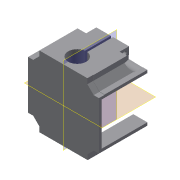
# Autodesk Inventor part: 20_Cube_insert_AlliedVision_Alvium_v3
Saved by Autodesk Inventor 2022 (Build 260153000, 153)
## iProperties
Created: 2019-08-07
Part Number: 20_Cube_insert_AlliedVision_Alvium_v3
Material: Generic
Document SubType Name: Modeling
Designer: marsikovabarbora
Density: 1 g/cm^3
Appearance: Default
Sheet Metal Rule: Standard
Author: marsikovabarbora
Autodesk Inventor part; units mm, degrees
ref_plane "Work Plane1" through (-29.1, -14.5, 2.4) normal (0, 0, -1) x (0, 1, 0)
ref_plane "Work Plane2" through (-13.8999, -10.5497, 2.25) normal (0, 0, -1) x (0, 1, 0)
ref_plane "Work Plane4" through (-17.3325, -17.0101, 2.3331) normal (0.0023441, 0.0023441, -0.9999945) x (-0.0000027, 0.9999973, 0.0023441)
sketch "Sketch1" plane through (0, 0, 0) normal (0, 0, 1) x (1, 0, 0)
  line L0 (-34.86, 0) -> (34.86, 0) construction
  line L1 (0, -34.86) -> (0, 34.86) construction
  line L2 (0, 0) -> (11.1575, 11.1575) construction
  line L3 (0, 0) -> (15.7791, 0) construction
  line L4 (0, 24.9) -> (16.8009, 24.9)
  line L5 (16.8009, 24.9) -> (16.8009, 21.2415)
  line L6 (16.8009, 21.2415) -> (19.0212, 19.0212)
  line L7 (24.9, 0) -> (24.9, 16.8009)
  line L8 (24.9, 16.8009) -> (21.2415, 16.8009)
  line L9 (21.2415, 16.8009) -> (19.0212, 19.0212)
  line L10 (0, -24.9) -> (16.8009, -24.9)
  line L11 (16.8009, -24.9) -> (16.8009, -21.2415)
  line L12 (16.8009, -21.2415) -> (19.0212, -19.0212)
  line L13 (24.9, 0) -> (24.9, -16.8009)
  line L14 (24.9, -16.8009) -> (21.2415, -16.8009)
  line L15 (21.2415, -16.8009) -> (19.0212, -19.0212)
  line L16 (0, 24.9) -> (-16.8009, 24.9)
  line L17 (-16.8009, 24.9) -> (-16.8009, 21.2415)
  line L18 (-16.8009, 21.2415) -> (-19.0212, 19.0212)
  line L19 (-24.9, 16.8009) -> (-21.2415, 16.8009)
  line L20 (-21.2415, 16.8009) -> (-19.0212, 19.0212)
  line L21 (0, -24.9) -> (-16.8009, -24.9)
  line L22 (-16.8009, -24.9) -> (-16.8009, -21.2415)
  line L23 (-16.8009, -21.2415) -> (-19.0212, -19.0212)
  line L24 (-21.2415, -16.8009) -> (-19.0212, -19.0212)
  line L25 (-24.9, -16.8009) -> (-21.2415, -16.8009)
  line L26 (-24.9, 0) -> (-24.9, -16.8009)
  line L27 (-24.9, 0) -> (-24.9, 16.8009)
  circle A0 centre (0, 0) radius 10
  dimension "d0" = 45
  dimension "d2" = 24.9
  dimension "d3" = 3.14
  dimension "d4" = 26.9
  dimension "d5" = 20
  constraints: 52 end point, 20 symmetric about line, 2 horizontal, 2 perpendicular, 2 point on line, 1 centre point, 1 coincident, 1 equal length
  measures "d0" angle of L3 L2
  measures "d2" distance between parallel lines of L0 L4
  measures "d3" distance of L5.end L6.end
  measures "d4" distance from line of L2.start L6
  measures "d5" diameter of A0
extrude "Extrusion1" add sketch "Sketch1" along normal blind 4 contours L4 L5 L6 L9 L8 L7 L13 L14 L15 L12 L11 L10 L21 L22 L23 L24 L25 L26 L27 L19 L20 L18 L17 L16 | A0
sketch "Skizze6" plane through (-16.8009, 24.9, 4) normal (0, 0, 1) x (1, 0, 0)
  circle A0 centre (6.8009, -18) radius 1.65 construction
  circle A1 centre (3.0009, -24.9) radius 1.65 construction
  circle A2 centre (26.5009, -34.9) radius 1.65 construction
  circle A3 centre (26.5009, -14.9) radius 1.65 construction
  line L0 (33.6017, -3.6585) -> (33.6017, 0) projected
  line L1 (33.6017, 0) -> (0, 0) construction
  line L2 (0, 0) -> (0, -3.6585) projected
  line L3 (0, -3.6585) -> (-4.4406, -8.0991) projected
  line L4 (-4.4406, -8.0991) -> (-8.0991, -8.0991) projected
  line L5 (-8.0991, -8.0991) -> (-8.0991, -41.7009) construction
  line L6 (-8.0991, -41.7009) -> (-4.4406, -41.7009) projected
  line L7 (-4.4406, -41.7009) -> (0, -46.1415) projected
  line L8 (0, -46.1415) -> (0, -49.8) projected
  line L9 (0, -49.8) -> (33.6017, -49.8) construction
  line L10 (33.6017, -49.8) -> (33.6017, -46.1415) projected
  line L11 (33.6017, -46.1415) -> (38.0423, -41.7009) projected
  line L12 (38.0423, -41.7009) -> (41.7009, -41.7009) projected
  line L13 (41.7009, -41.7009) -> (41.7009, -8.0991) construction
  line L14 (41.7009, -8.0991) -> (38.0423, -8.0991) projected
  line L15 (38.0423, -8.0991) -> (33.6017, -3.6585) projected
  line L16 (-0.2, 0.2) -> (33.8017, 0.2) construction
  line L17 (33.8017, 0.2) -> (33.8017, -3.5757)
  line L18 (33.8017, -3.5757) -> (38.1252, -7.8991)
  line L19 (38.1252, -7.8991) -> (41.9009, -7.8991)
  line L20 (41.9009, -7.8991) -> (41.9009, -41.9009) construction
  line L21 (41.9009, -41.9009) -> (38.1252, -41.9009)
  line L22 (38.1252, -41.9009) -> (33.8017, -46.2243)
  line L23 (33.8017, -46.2243) -> (33.8017, -50)
  line L24 (33.8017, -50) -> (-0.2, -50) construction
  line L25 (-0.2, -50) -> (-0.2, -46.2243)
  line L26 (-0.2, -46.2243) -> (-4.5235, -41.9009)
  line L27 (-4.5235, -41.9009) -> (-8.2991, -41.9009)
  line L28 (-8.2991, -41.9009) -> (-8.2991, -7.8991) construction
  line L29 (-8.2991, -7.8991) -> (-4.5235, -7.8991)
  line L30 (-4.5235, -7.8991) -> (-0.2, -3.5757)
  line L31 (-0.2, -3.5757) -> (-0.2, 0.2)
  line L32 (-8.0991, -8.0991) -> (-8.0991, -7.8991)
  line L33 (0, 0) -> (-0.2, 0)
  line L34 (33.6017, 0) -> (33.8017, 0)
  line L35 (41.7009, -8.0991) -> (38.0423, -8.0991) projected
  line L36 (41.7009, -8.0991) -> (41.7009, -7.8991)
  line L37 (41.7009, -41.7009) -> (41.7009, -41.9009)
  line L38 (33.6017, -49.8) -> (33.8017, -49.8)
  line L39 (-8.0991, -41.7009) -> (-8.0991, -41.9009)
  line L40 (0, -49.8) -> (-0.2, -49.8)
  point P0 (16.8009, -24.9)
  dimension "d25" = 0.2
  constraints: 48 end point, 12 point on line, 4 perpendicular, 15 other
  measures "d25" distance between parallel lines of L1 L16
extrude "IM_offset" add sketch "Skizze6" against normal up to surface (4 mm away) contours L2 L3 L4 L32 L29 L30 L31 L33 | L6 L7 L8 L40 L25 L26 L27 L39 | L10 L11 L12 L37 L21 L22 L23 L38
ref_plane "Work Plane3" through (-24.85, -16.97, -31.85) normal (0, 0, 1) x (1, 0, 0)
sketch "Sketch9" plane through (0, 0, 0) normal (0, 0, -1) x (-1, 0, 0)
  line L0 (21.2829, 16.9009) -> (17.0009, 21.2829)
  line L1 (17.0009, 21.2829) -> (17.0009, 24.9)
  line L2 (24.9, 17.0009) -> (21.2829, 16.9009)
  line L3 (24.9, -17.0009) -> (24.9, 17.0009) projected
  line L4 (17.0009, 24.9) -> (-16.8009, 24.9) projected
  line L5 (24.9, 14.96) -> (15.0009, 14.96)
  line L6 (15.0009, 14.96) -> (15.0009, 24.9)
  line L7 (15.0009, 24.9) -> (17.0009, 24.9)
  line L8 (24.9, 17.0009) -> (24.9, 14.96)
  line L9 (-16.9009, 21.2829) -> (-21.2829, 17.0009)
  line L10 (-21.2829, 17.0009) -> (-24.9, 17.0009)
  line L11 (-17.0009, 24.9) -> (-16.9009, 21.2829)
  line L12 (-14.96, 24.9) -> (-14.96, 15.0009)
  line L13 (-14.96, 15.0009) -> (-24.9, 15.0009)
  line L14 (-24.9, 15.0009) -> (-24.9, 17.0009)
  line L15 (-17.0009, 24.9) -> (-14.96, 24.9)
  line L16 (-21.2829, -16.9009) -> (-17.0009, -21.2829)
  line L17 (-17.0009, -21.2829) -> (-17.0009, -24.9)
  line L18 (-24.9, -17.0009) -> (-21.2829, -16.9009)
  line L19 (-24.9, -14.96) -> (-15.0009, -14.96)
  line L20 (-15.0009, -14.96) -> (-15.0009, -24.9)
  line L21 (-15.0009, -24.9) -> (-17.0009, -24.9)
  line L22 (-24.9, -17.0009) -> (-24.9, -14.96)
  line L23 (16.9009, -21.2829) -> (21.2829, -17.0009)
  line L24 (21.2829, -17.0009) -> (24.9, -17.0009)
  line L25 (17.0009, -24.9) -> (16.9009, -21.2829)
  line L26 (14.96, -24.9) -> (14.96, -15.0009)
  line L27 (14.96, -15.0009) -> (24.9, -15.0009)
  line L28 (24.9, -15.0009) -> (24.9, -17.0009)
  line L29 (17.0009, -24.9) -> (14.96, -24.9)
  point P0 (0, 0)
  dimension "d44" = 2
  dimension "d47" = 360
  constraints: 56 end point, 10 point on line, 2 parallel, 1 horizontal, 1 perpendicular, 65 other
  measures "d44" distance of L6.end L7.end
ref_plane "Work Plane5" through (-25.1325, -16.9302, -31.7852) normal (-0.0023441, -0.0023441, 0.9999945) x (0.9999973, -0.0000027, 0.0023441)
ref_plane "Work Plane10" through (-16.97, -16.97, -30.1) normal (0, 0, 1) x (1, 0, 0)
extrude "Extrusion9" add sketch "Sketch9" along normal up to surface (30.1 mm away)
ref_plane "Work Plane6" through (-16.5464, -17.0101, 2.3349) normal (0.0023441, 0.0023441, -0.9999945) x (-0.0000027, 0.9999973, 0.0023441)
sketch "Sketch11" plane through (0, 0, 4) normal (0, 0, 1) x (1, 0, 0)
  circle A0 centre (-10, 6.9) radius 1.65 projected
  circle A1 centre (9.7, 10) radius 1.65 projected
  circle A2 centre (9.7, -10) radius 1.65 projected
  arc A3 (-13.0126, 1.45) -> (-13.0126, -1.45) centre (-13.8, 0) ccw projected
  line L0 (-13.0126, 1.45) -> (15.2888, 1.45) projected
  line L1 (15.2888, -1.45) -> (-13.0126, -1.45) projected
  arc A4 (15.2888, -1.45) -> (15.2888, 1.45) centre (16.0762, 0) ccw projected
  line L2 (16.8009, 24.9) -> (-17.0009, 24.9) projected
  line L3 (-17.0009, 24.9) -> (-17.0009, 21.3243) projected
  line L4 (-17.0009, 21.3243) -> (-21.3243, 17.0009) projected
  line L5 (-21.3243, 17.0009) -> (-24.9, 17.0009) projected
  line L6 (-24.9, 17.0009) -> (-24.9, -17.0009) projected
  line L7 (-24.9, -17.0009) -> (-21.3243, -17.0009) projected
  line L8 (-21.3243, -17.0009) -> (-17.0009, -21.3243) projected
  line L9 (-17.0009, -21.3243) -> (-17.0009, -24.9) projected
  line L10 (-17.0009, -24.9) -> (17.0009, -24.9) projected
  line L11 (17.0009, -24.9) -> (17.0009, -21.3243) projected
  line L12 (17.0009, -21.3243) -> (21.3243, -17.0009) projected
  line L13 (21.3243, -17.0009) -> (24.9, -17.0009) projected
  line L14 (24.9, -17.0009) -> (24.9, 16.8009) projected
  line L15 (24.9, 16.8009) -> (21.2415, 16.8009) projected
  line L16 (21.2415, 16.8009) -> (16.8009, 21.2415) projected
  line L17 (16.8009, 21.2415) -> (16.8009, 24.9) projected
  point P0 (0, 0)
ref_plane "Work Plane7" through (-24.4263, -24.8901, 2.298) normal (0.0023441, 0.0023441, -0.9999945) x (-0.0000027, 0.9999973, 0.0023441)
extrude "Extrusion11" add sketch "Sketch11" against normal up to surface surface through (-24.4263, -24.8901, 2.298) normal (0.0023441, 0.0023441, -0.9999945)
ref_plane "Work Plane8" through (-15.0009, 0, 0) normal (0, 1, 0) x (1, 0, 0)
ref_plane "Work Plane9" through (0, -15.0009, 0) normal (-1, 0, 0) x (0, 0, 1)
sketch "Sketch12" plane through (-24.9, -17.0009, 4) normal (-1, 0, 0) x (0, 0, 1)
  line L0 (0, 34.0017) -> (-4, 34.0017) projected
  line L1 (-4, 34.0017) -> (-34.1, 34.0017) projected
  line L2 (-34.1, 31.9609) -> (-34.1, 34.0017) projected
  line L3 (-4, 31.9609) -> (-34.1, 31.9609) projected
  line L4 (-4, 2) -> (-4, 31.9609) projected
  line L5 (-4, 2) -> (-34.1, 2) projected
  line L6 (-34.1, 0) -> (-34.1, 2) projected
  line L7 (0, 0) -> (-34.1, 0) projected
  line L8 (0, 34.0017) -> (0, 0) projected
  line L9 (-4, 32.0017) -> (-34.1, 32.0017) projected
  line L10 (-34.1, 2) -> (-34.1, -7.8991) projected
  line L11 (-34.1, 32.0017) -> (-34.1, 2)
  line L12 (-4, 31.9609) -> (-34.1, 31.9609)
  line L13 (-34.1, 31.9609) -> (-34.1, 2)
  line L14 (-34.1, 2) -> (-4, 2)
  line L15 (-4, 2) -> (-4, 31.9609)
  circle A0 centre (-17.13, 17.0009) radius 6.35
  dimension "d102" = 12.7
  constraints: 10 end point, 2 parallel, 1 centre point, 1 horizontal, 1 perpendicular, 1 other
  measures "d102" diameter of A0
extrude "Extrusion12" add sketch "Sketch12" against normal up to surface (9.94 mm away) contours L11 L3 L4 L5
sketch "Sketch14" plane through (-24.9, -17.0009, 4) normal (0, -1, 0) x (1, 0, 0)
  line L0 (0, -31.2951) -> (0, -13.7755) projected
  line L1 (3.6171, -34.1) -> (0, -34.1) projected
  point P0 (24.9, -4)
  point P1 (0, -31.2915)
  point P2 (3, -31.1)
  dimension "d71" = 3
  dimension "d72" = 3
  measures "d71" distance from line of L1 point (3, -31.1)
  measures "d72" distance from line of L0 point (3, -31.1)
hole "Hole2" at (-21.9, -17.0009, -27.1) direction (0, 1, 0) diameter 2.9 end through all counterbore diameter 6 counterbore depth 3
sketch "Sketch15" plane through (-24.9, -17.0009, 4) normal (0, -1, 0) x (1, 0, 0)
  arc A0 (3.6171, -28.1642) -> (3.6171, -34.0358) centre (3, -31.1) ccw projected
  circle A1 centre (3, -31.1) radius 3
  arc A2 (4.0578, -26.0674) -> (3.4649, -36.2215) centre (3, -31.1) ccw
  circle A3 centre (3, -31.1) radius 5.1426
  point P0 (24.9, -4)
  point P1 (0.0578, -35.7847)
  constraints: 2 centre point, 2 coincident, 2 point on circle, 1 concentric, 3 other
extrude "Extrusion14" cut sketch "Sketch15" along normal blind 10 and the other way blind 6 contours A1 A0 | A3 A2
sketch "Sketch16" plane through (-24.9, 17.0009, 0) normal (0.027636, 0.9996181, 0) x (0.9996181, -0.027636, 0)
  ellipse E0 centre (3.0011, 27.1) end of major axis (4.4517, 27.1) minor radius 1.45 (3.6185, 28.4121) -> (3.6185, 25.7879) ccw projected
  ellipse E1 centre (3.7727, 27.1) end of major axis (3.7727, 21.9574) minor radius 5.1406 (0.7739, 22.9232) -> (7.9479, 30.1) ccw projected
  circle A0 centre (3.7727, 27.1) radius 5.1426
  point P0 (25.3603, 0)
  constraints: 1 centre point, 1 coincident, 3 other
extrude "Extrusion15" cut sketch "Sketch16" along normal mid plane 10
sketch "Sketch17" plane through (-17.0009, 24.9, 4) normal (0, 1, 0) x (1, 0, 0)
  line L0 (33.8017, 4) -> (33.8017, 0) projected
  line L1 (33.8017, 4) -> (34.0017, 4) projected
  line L2 (34.0017, 4) -> (34.0017, 34.1) projected
  line L3 (31.9609, 34.1) -> (34.0017, 34.1) projected
  line L4 (31.9609, 4) -> (31.9609, 34.1) projected
  line L5 (2, 4) -> (31.9609, 4) projected
  line L6 (2, 4) -> (2, 34.1) projected
  line L7 (0, 34.1) -> (2, 34.1) projected
  line L8 (0, 0) -> (0, 34.1) projected
  line L9 (33.8017, 0) -> (0, 0) projected
  line L10 (0, 34.1) -> (2, 34.1) projected
  line L11 (2, 34.1) -> (31.9609, 34.1)
  line L12 (31.9609, 34.1) -> (31.9609, 4)
  line L13 (31.9609, 4) -> (2, 4)
  line L14 (2, 4) -> (2, 34.1)
  circle A0 centre (17.0009, 9.63) radius 6.35
  point P0 (17.0009, 4)
  point P1 (14.0639, 4)
  point P2 (19.9378, 4)
  dimension "d103" = 12.7
  constraints: 8 end point, 2 parallel, 1 centre point, 1 horizontal, 1 perpendicular, 1 other
  measures "d103" diameter of A0
extrude "Extrusion16" add sketch "Sketch17" against normal up to surface (9.8991 mm away) contours L4 L5 A0 L6 L11
sketch "Sketch18" plane through (0, 0, 0) normal (0, 0, -1) x (-1, 0, 0)
  line L0 (-16.8009, 24.9) -> (17.0009, 24.9) projected
  line L1 (17.0009, 24.9) -> (17.0009, 21.3243) projected
  line L2 (17.0009, 21.3243) -> (21.3243, 17.0009) projected
  line L3 (21.3243, 17.0009) -> (24.9, 17.0009) projected
  line L4 (24.9, 17.0009) -> (24.9, -17.0009) projected
  line L5 (24.9, -17.0009) -> (21.3243, -17.0009) projected
  line L6 (21.3243, -17.0009) -> (17.0009, -21.3243) projected
  line L7 (17.0009, -21.3243) -> (17.0009, -24.9) projected
  line L8 (17.0009, -24.9) -> (-17.0009, -24.9) projected
  line L9 (-17.0009, -24.9) -> (-17.0009, -21.3243) projected
  line L10 (-17.0009, -21.3243) -> (-21.3243, -17.0009) projected
  line L11 (-21.3243, -17.0009) -> (-24.9, -17.0009) projected
  line L12 (-24.9, -17.0009) -> (-24.9, 16.8009) projected
  line L13 (-24.9, 16.8009) -> (-21.2415, 16.8009) projected
  line L14 (-21.2415, 16.8009) -> (-16.8009, 21.2415) projected
  line L15 (-16.8009, 21.2415) -> (-16.8009, 24.9) projected
  circle A0 centre (0, 0) radius 0.5
  point P0 (0, 0)
  dimension "d79" = 1
  constraints: 1 centre point
  measures "d79" diameter of A0
extrude "Extrusion17" cut sketch "Sketch18" against normal through all contours A0
pattern_circular "Circular Pattern1" count 2 over 90 about axis through (0, 0, 0) along (0, 0, -1) of "Hole2", "Extrusion14", "Extrusion15"
sketch "Sketch19" plane through (-17.0009, 24.9, 4) normal (0, 1, 0) x (1, 0, 0)
  line L0 (17.7509, 38.7619) -> (16.2509, 38.7619)
  line L1 (16.2509, 38.7619) -> (16.2509, 17.8739)
  line L2 (16.2509, 17.8739) -> (17.7509, 17.8739)
  line L3 (17.7509, 17.8739) -> (17.7509, 38.7619)
  line L4 (17.7509, 38.7619) -> (16.2509, 17.8739) construction
  line L5 (16.2509, 38.7619) -> (17.7509, 17.8739) construction
  line L6 (16.2509, 17.8739) -> (17.7509, 17.8739)
  line L7 (17.7509, 17.8739) -> (17.7509, 13.2168)
  line L8 (17.7509, 13.2168) -> (16.2509, 13.2168)
  line L9 (16.2509, 13.2168) -> (16.2509, 17.8739)
  point P0 (17.0009, 4)
  point P1 (17.0009, 28.3179)
  dimension "d85" = 1.5
  constraints: 20 end point, 4 parallel, 2 horizontal, 2 midpoint, 2 perpendicular
  measures "d85" distance of L2.end L1.end
extrude "Extrusion18" cut sketch "Sketch19" against normal blind 10
sketch "Sketch20" plane through (-14.96, -24.9, -30.1) normal (0, 0, -1) x (-1, 0, 0)
  line L0 (9.94, 31.25) -> (9.94, 18.55) projected
  line L1 (9.94, 24.9) -> (0, 24.9)
  line L2 (0, 39.86) -> (0, 0) projected
  line L3 (4.97, 24.9) -> (4.97, 24.1)
  line L4 (0, 25.7) -> (9.94, 25.7)
  line L5 (9.94, 25.7) -> (9.94, 24.1)
  line L6 (9.94, 24.1) -> (0, 24.1)
  line L7 (0, 24.1) -> (0, 25.7)
  line L8 (0, 25.7) -> (9.94, 24.1) construction
  line L9 (9.94, 25.7) -> (0, 24.1) construction
  point P0 (-14.96, 24.9)
  point P1 (0, 24.1)
  point P2 (9.94, 24.1)
  point P3 (9.94, 25.7)
  point P4 (0, 25.7)
  dimension "d93" = 0.8
  constraints: 16 end point, 4 midpoint, 2 parallel, 2 perpendicular, 1 horizontal, 1 point on line, 1 vertical
  measures "d93" distance of L3.start L3.end
extrude "Extrusion19" cut sketch "Sketch20" against normal up to surface
sketch "Sketch22" plane through (0, 0, 0) normal (0, 0, -1) x (-1, 0, 0)
  line L0 (-24.9, 15.0009) -> (-24.9, -14.96) projected
  line L1 (-24.9, -14.96) -> (-15.0009, -14.96) projected
  line L2 (-15.0009, -14.96) -> (-15.0009, -24.9) projected
  line L3 (-15.0009, -24.9) -> (14.96, -24.9) projected
  line L4 (14.96, -24.9) -> (14.96, 14.96)
  line L5 (14.96, 15.0009) -> (2.9369, 15.0009)
  line L6 (14.96, 14.96) -> (14.96, 15.0009)
  line L7 (2.9369, 15.0009) -> (2.9369, 24.9) projected
  line L8 (2.9369, 15.0009) -> (-24.9, 15.0009)
  point P0 (0, 0)
  constraints: 8 end point, 1 perpendicular
extrude "Extrusion20" cut sketch "Sketch22" against normal blind 2
sketch "Sketch23" plane through (-17.0009, 24.9, 4) normal (0, 1, 0) x (1, 0, 0)
  circle A0 centre (17.0009, 9.63) radius 6.475 construction
  circle A1 centre (17.0009, 9.63) radius 6.35
  point P0 (17.0009, 4)
  dimension "d104" = 12.7
  constraints: 2 centre point, 2 other
  measures "d104" diameter of A1
extrude "Extrusion21" cut sketch "Sketch23" against normal through all
equation "\"GapSize\" = Thickness"
equation "\"BendRadius\" = Thickness"
equation "\"MinimumRemnant\" = 2 * Thickness"
equation "\"BendReliefDepth\" = 0.5 * Thickness"
equation "\"BendReliefWidth\" = Thickness"
equation "\"CornerReliefSize\" = 4 * Thickness"
equation "\"JacobiRadiusSize\" = Thickness"
equation "\"TransitionRadius\" = BendRadius"
equation "\"Thickness\" = 0.5"
body "Solid1"
